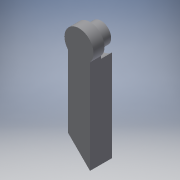
# Autodesk Inventor part: Latch
Saved by Autodesk Inventor 2019 (Build 230136000, 136)
## iProperties
Created: 2018-08-02
Part Number: Latch
Material: Generic
Document SubType Name: Modeling
Designer: zacha
Density: 1 g/cm^3
Appearance: Default
Author: zacha
Autodesk Inventor part; units mm, degrees
ref_plane "YZ Plane" through (0, 0, 0) normal (1, 0, 0) x (0, 1, 0)
ref_plane "XZ Plane" through (0, 0, 0) normal (0, 1, 0) x (-1, 0, 0)
ref_plane "XY Plane" through (0, 0, 0) normal (0, 0, 1) x (1, 0, 0)
sketch "Sketch3" plane through (0, 0, 0) normal (0, 0, 1) x (1, 0, 0)
  circle A0 centre (14.5794, 0.9769) radius 3.175 projected
  arc A1 (14.5794, -3.4681) -> (19.0244, 0.9769) centre (14.5794, 0.9769) ccw projected
  line L0 (19.0244, 5.4219) -> (19.0244, 0.9769) projected
  line L1 (14.5794, 5.4219) -> (19.0244, 5.4219) projected
  arc A2 (14.5794, 5.4219) -> (10.1344, 0.9769) centre (14.5794, 0.9769) ccw projected
  line L2 (10.1344, -3.4681) -> (10.1344, 0.9769) projected
  line L3 (14.5794, -3.4681) -> (10.1344, -3.4681) projected
  circle A3 centre (14.5794, 0.9769) radius 2.921
  point P0 (0, 0)
  dimension "d3" = 5.842
  constraints: 1 centre point, 1 coincident
  measures "d3" diameter of A3
extrude "Extrusion2" add sketch "Sketch3" against normal blind 6.35 contours A3
sketch "Sketch4" plane through (14.5794, 0.9769, 0) normal (0, 0, 1) x (1, 0, 0)
  circle A0 centre (0, 0) radius 4.191
  circle A1 centre (0, 0) radius 3.175 projected
  arc A2 (0, -4.445) -> (4.445, 0) centre (0, 0) ccw projected
  line L0 (4.445, 4.445) -> (4.445, 0) projected
  line L1 (0, 4.445) -> (4.445, 4.445) projected
  arc A3 (0, 4.445) -> (-4.445, 0) centre (0, 0) ccw projected
  line L2 (-4.445, -4.445) -> (-4.445, 0) projected
  line L3 (0, -4.445) -> (-4.445, -4.445) projected
  circle A4 centre (0, 0) radius 2.921 projected
  point P0 (-14.5794, -0.9769)
  dimension "d6" = 8.382
  constraints: 1 centre point, 1 concentric
  measures "d6" diameter of A0
extrude "Extrusion3" add sketch "Sketch4" against normal blind 3.175 contours A0 | A1 | A4
sketch "Sketch5" plane through (14.5794, 0.9769, 0) normal (0, 0, 1) x (1, 0, 0)
  circle A0 centre (0, 0) radius 4.191 projected
  line L0 (-3.175, -23.495) -> (-3.175, 0)
  line L1 (-3.175, -23.495) -> (3.175, -29.845)
  line L2 (3.175, -29.845) -> (3.175, 0)
  circle A1 centre (0, 0) radius 3.175
  line L3 (3.175, -29.845) -> (-3.175, -23.495) projected
  point P0 (-14.5794, -0.9769)
  dimension "d9" = 6.35
  constraints: 6 end point, 2 point on circle, 2 vertical, 1 centre point, 1 coincident
  measures "d9" diameter of A1
extrude "Extrusion4" add sketch "Sketch5" against normal blind 3.175 contours L0 A1 L2 A0 | A0 L2 L1 L0 picked at (0.1276, -3.8236)
sketch "Sketch6" plane through (14.5794, 0.9769, -3.175) normal (0, 0, -1) x (-1, 0, 0)
  arc A0 (-4.445, 0) -> (0, -4.445) centre (0, 0) ccw projected
  line L0 (0, -4.445) -> (23.405, -4.445) projected
  line L1 (-3.175, -2.7357) -> (-3.175, -29.845) projected
  line L2 (3.175, -2.7357) -> (3.175, -23.495) projected
  line L3 (-3.175, -29.845) -> (3.175, -23.495)
  line L4 (3.175, -23.495) -> (3.175, -4.699)
  line L5 (-3.175, -3.4641) -> (-3.175, -29.845)
  arc A1 (0, -4.699) -> (-3.175, -3.4641) centre (0, 0) ccw construction
  line L6 (0, -4.699) -> (3.175, -4.699)
  arc A2 (-3.175, -3.4641) -> (0, -4.699) centre (0, 0) ccw
  point P0 (14.5794, -0.9769)
  dimension "d12" = 9.398
  constraints: 8 end point, 4 point on circle, 2 centre point, 2 point on line, 1 coincident, 1 parallel, 1 perpendicular, 1 tangent
  measures "d12" diameter of A1
extrude "Extrusion5" add sketch "Sketch6" along normal blind 3.175 contours A2 L6 L2 L3 L1
body "Solid2"
